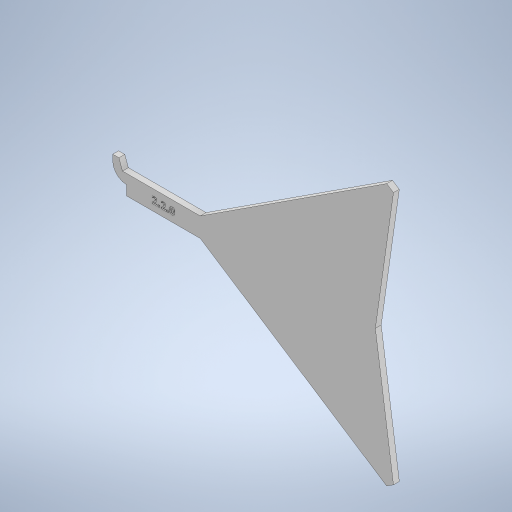
# Autodesk Inventor part: WindFinAlt
Saved by Autodesk Inventor 2024.3 (Build 283343000, 343)
## iProperties
Created: 2025-01-27
Part Number: WindFinAlt
Material: Generisch
Document SubType Name: Modeling
Designer: Maximilian Hock
Density: 1 g/cm^3
Appearance: Vorgabe
Author: Maximilian Hock
## iProperties of the stored document WindFinAlt_3D-Druck.ipt
Created: 2025-01-27
Part Number: WindFinAlt_3D-Druck
Material: Generisch
Document SubType Name: Modeling
Designer: Maximilian Hock
Density: 1 g/cm^3
Appearance: Vorgabe
Author: Maximilian Hock
Autodesk Inventor part; units mm, degrees
ref_plane "YZ Plane" through (0, 0, 0) normal (1, 0, 0) x (0, 1, 0)
ref_plane "XZ Plane" through (0, 0, 0) normal (0, 1, 0) x (-1, 0, 0)
ref_plane "XY Plane" through (0, 0, 0) normal (0, 0, 1) x (1, 0, 0)
sketch "Skizze1" plane through (0, 0, 0) normal (0, 1, 0) x (-1, 0, 0)
  line L0 (0, 0) -> (0, 5)
  line L1 (0, 5) -> (5, 5)
  line L2 (5, 5) -> (5, 0)
  line L3 (0, 0) -> (-40, 0)
  line L4 (-2, -5) -> (-2, -10)
  line L5 (-140, -75) -> (-130, -5)
  line L6 (-130, -5) -> (-140, 65)
  line L7 (-140, 65) -> (-40, 0)
  line L8 (0, -5) -> (-2, -5)
  line L9 (-2, -10) -> (-40, -10)
  line L10 (-40, -10) -> (-140, -75)
  line L11 (-40, -10) -> (-40, 0)
  arc A0 (0, -5) -> (5, 0) centre (0, 0) ccw
  arc A1 (-2, -5) -> (5, 2) centre (-2, 2) ccw
  line L12 (0, 0) -> (1.8199, 5)
  point P0 (-40, -5)
  dimension "d2" = 100
  dimension "d3" = 5
  dimension "d4" = 140
  dimension "d5" = 10
  dimension "d6" = 140
  dimension "d7" = 2
  dimension "d13" = 20
  constraints: 26 end point, 4 equal length, 4 point on circle, 4 tangent, 3 horizontal, 3 point on line, 3 vertical, 2 centre point, 2 perpendicular, 1 coincident, 1 horizontal alignment, 1 midpoint
  measures "d2" horizontal distance of L6.end L3.end
  measures "d3" distance of L4.start L4.end
  measures "d4" distance of L5.start L6.end
  measures "d5" horizontal distance of L6.end L5.end
  measures "d6" horizontal distance of L6.end L0.start
  measures "d7" distance between parallel lines of L4 L0
  measures "d13" angle of L0 L12
extrude "Extrusion1" add sketch "Skizze1" along normal blind 3 contours L12 L1 L2 A1 L4 L9 L11 L3 | L11 L10 L5 L6 L7
chamfer "Fasen1" distance 5 angle 45 2 edges at (140, 1.5, 65) (140, 1.5, -75)
sketch "Skizze2" plane through (0, 0, 0) normal (0, -1, 0) x (1, 0, 0)
  line L0 (2, 0) -> (40, 0) construction
  line L1 (40, 0) -> (40, -10) construction
  line L2 (40, -10) -> (2, -10) construction
  line L3 (2, -10) -> (2, 0) construction
  line L4 (17.8248, -6.7486) -> (15.2522, -6.7486)
  line L5 (15.2522, -6.7486) -> (15.2522, -6.1785)
  spline S0 degree 2 poles (15.2522, -6.1785) (15.5784, -5.9175) (16.1003, -5.4581) (16.296, -5.251) knots 0 0 0 1 2 2 2
  spline S1 degree 2 poles (16.296, -5.251) (16.5541, -4.9816) (16.7838, -4.5703) (16.7838, -4.3547) knots 0 0 0 1 2 2 2
  spline S2 degree 2 poles (16.7838, -4.3547) (16.7838, -4.1108) (16.4917, -3.8499) (16.2308, -3.8499) knots 0 0 0 1 2 2 2
  spline S3 degree 2 poles (16.2308, -3.8499) (16.0974, -3.8499) (15.8592, -3.9151) (15.7372, -3.9662) knots 0 0 0 1 2 2 2
  spline S4 degree 2 poles (15.7372, -3.9662) (15.6181, -4.0201) (15.4479, -4.1335) (15.4054, -4.1619) knots 0 0 0 1 2 2 2
  line L6 (15.4054, -4.1619) -> (15.3373, -4.1619)
  line L7 (15.3373, -4.1619) -> (15.3373, -3.3989)
  spline S5 degree 2 poles (15.3373, -3.3989) (15.4848, -3.328) (16.1145, -3.1805) (16.4066, -3.1805) knots 0 0 0 1 2 2 2
  spline S6 degree 2 poles (16.4066, -3.1805) (17.0306, -3.1805) (17.6716, -3.7364) (17.6716, -4.2385) knots 0 0 0 1 2 2 2
  spline S7 degree 2 poles (17.6716, -4.2385) (17.6716, -4.5476) (17.3795, -5.1432) (17.0419, -5.4836) knots 0 0 0 1 2 2 2
  spline S8 degree 2 poles (17.0419, -5.4836) (16.8292, -5.6935) (16.4293, -6.0197) (16.3414, -6.0877) knots 0 0 0 1 2 2 2
  line L8 (16.3414, -6.0877) -> (17.8248, -6.0877)
  line L9 (17.8248, -6.0877) -> (17.8248, -6.7486)
  line L10 (19.1295, -6.7486) -> (18.2984, -6.7486)
  line L11 (18.2984, -6.7486) -> (18.2984, -5.8239)
  line L12 (18.2984, -5.8239) -> (19.1295, -5.8239)
  line L13 (19.1295, -5.8239) -> (19.1295, -6.7486)
  line L14 (22.394, -6.7486) -> (19.8215, -6.7486)
  line L15 (19.8215, -6.7486) -> (19.8215, -6.1785)
  spline S9 degree 2 poles (19.8215, -6.1785) (20.1477, -5.9175) (20.6696, -5.4581) (20.8653, -5.251) knots 0 0 0 1 2 2 2
  spline S10 degree 2 poles (20.8653, -5.251) (21.1234, -4.9816) (21.3531, -4.5703) (21.3531, -4.3547) knots 0 0 0 1 2 2 2
  spline S11 degree 2 poles (21.3531, -4.3547) (21.3531, -4.1108) (21.061, -3.8499) (20.8, -3.8499) knots 0 0 0 1 2 2 2
  spline S12 degree 2 poles (20.8, -3.8499) (20.6667, -3.8499) (20.4285, -3.9151) (20.3065, -3.9662) knots 0 0 0 1 2 2 2
  spline S13 degree 2 poles (20.3065, -3.9662) (20.1874, -4.0201) (20.0172, -4.1335) (19.9747, -4.1619) knots 0 0 0 1 2 2 2
  line L16 (19.9747, -4.1619) -> (19.9066, -4.1619)
  line L17 (19.9066, -4.1619) -> (19.9066, -3.3989)
  spline S14 degree 2 poles (19.9066, -3.3989) (20.0541, -3.328) (20.6838, -3.1805) (20.9759, -3.1805) knots 0 0 0 1 2 2 2
  spline S15 degree 2 poles (20.9759, -3.1805) (21.5999, -3.1805) (22.2409, -3.7364) (22.2409, -4.2385) knots 0 0 0 1 2 2 2
  spline S16 degree 2 poles (22.2409, -4.2385) (22.2409, -4.5476) (21.9487, -5.1432) (21.6112, -5.4836) knots 0 0 0 1 2 2 2
  spline S17 degree 2 poles (21.6112, -5.4836) (21.3985, -5.6935) (20.9986, -6.0197) (20.9107, -6.0877) knots 0 0 0 1 2 2 2
  line L18 (20.9107, -6.0877) -> (22.394, -6.0877)
  line L19 (22.394, -6.0877) -> (22.394, -6.7486)
  line L20 (23.6987, -6.7486) -> (22.8677, -6.7486)
  line L21 (22.8677, -6.7486) -> (22.8677, -5.8239)
  line L22 (22.8677, -5.8239) -> (23.6987, -5.8239)
  line L23 (23.6987, -5.8239) -> (23.6987, -6.7486)
  spline S18 degree 2 poles (26.9179, -4.9986) (26.9179, -5.4524) (26.7733, -6.1331) (26.6116, -6.3628) knots 0 0 0 1 2 2 2
  spline S19 degree 2 poles (26.6116, -6.3628) (26.4528, -6.5897) (25.9394, -6.8223) (25.5707, -6.8223) knots 0 0 0 1 2 2 2
  spline S20 degree 2 poles (25.5707, -6.8223) (25.1991, -6.8223) (24.6886, -6.5897) (24.5269, -6.3572) knots 0 0 0 1 2 2 2
  spline S21 degree 2 poles (24.5269, -6.3572) (24.3653, -6.1274) (24.2206, -5.4524) (24.2206, -4.9986) knots 0 0 0 1 2 2 2
  spline S22 degree 2 poles (24.2206, -4.9986) (24.2206, -4.5334) (24.3653, -3.8754) (24.5298, -3.6372) knots 0 0 0 1 2 2 2
  spline S23 degree 2 poles (24.5298, -3.6372) (24.6943, -3.4046) (25.2133, -3.1777) (25.5707, -3.1777) knots 0 0 0 1 2 2 2
  spline S24 degree 2 poles (25.5707, -3.1777) (25.9479, -3.1777) (26.4528, -3.4159) (26.6145, -3.6513) knots 0 0 0 1 2 2 2
  spline S25 degree 2 poles (26.6145, -3.6513) (26.7733, -3.8811) (26.9179, -4.559) (26.9179, -4.9986) knots 0 0 0 1 2 2 2
  spline S26 degree 2 poles (26.0359, -4.9986) (26.0359, -4.3491) (25.8231, -3.8244) (25.5707, -3.8244) knots 0 0 0 1 2 2 2
  spline S27 degree 2 poles (25.5707, -3.8244) (25.3183, -3.8244) (25.1027, -4.3491) (25.1027, -5.0014) knots 0 0 0 1 2 2 2
  spline S28 degree 2 poles (25.1027, -5.0014) (25.1027, -5.6424) (25.3183, -6.1756) (25.5707, -6.1756) knots 0 0 0 1 2 2 2
  spline S29 degree 2 poles (25.5707, -6.1756) (25.8203, -6.1756) (26.0359, -5.6424) (26.0359, -4.9986) knots 0 0 0 1 2 2 2
  point P0 (0, 0)
  point P1 (2, -10)
  constraints: 2 coincident, 2 other
emboss "Prägen1" sketch "Skizze2" operation cut depth 0.5 direction (0, 1, 0)
equation "\"d0\" = FinThickness"
equation "\"FinThickness\" = 3"
